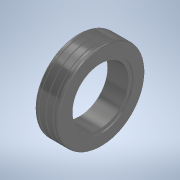
# Autodesk Inventor part: Wheel 75 mm - Part 1
Saved by Autodesk Inventor 2020 (Build 240168000, 168)
## iProperties
Created: 2023-01-26
Part Number: Wheel 75 mm - Part 1
Material: Generic
Document SubType Name: Modeling
Designer: saad.nashed
Density: 1 g/cm^3
Appearance: Rubber - Black - Version 1.1
d3: 24.000 mm
d4: 3.000 mm
d1: 20.250 mm
d5: 1.125 mm
d0: 37.500 mm
Author: saad.nashed
Autodesk Inventor part; units mm, degrees
ref_plane "YZ Plane" through (0, 0, 0) normal (1, 0, 0) x (0, 1, 0)
ref_plane "XZ Plane" through (0, 0, 0) normal (0, 1, 0) x (-1, 0, 0)
ref_plane "XY Plane" through (0, 0, 0) normal (0, 0, 1) x (1, 0, 0)
sketch "Sketch1" plane through (0, 0, 0) normal (0, 1, 0) x (-1, 0, 0)
  line L0 (13.955, 0) -> (0, 0) construction
  line L1 (0, 0) -> (0, -8.8012) construction
  line L2 (-9, -24) -> (9, -24)
  line L3 (9, -24) -> (9, -27)
  line L4 (9, -27) -> (10.125, -27)
  line L5 (10.125, -27) -> (10.125, -35.475)
  arc A0 (8.1, -37.5) -> (10.125, -35.475) centre (8.1, -35.475) ccw
  line L6 (8.1, -37.5) -> (-8.1, -37.5)
  arc A1 (-10.125, -35.475) -> (-8.1, -37.5) centre (-8.1, -35.475) ccw
  line L7 (-10.125, -35.475) -> (-10.125, -27)
  line L8 (-10.125, -27) -> (-9, -27)
  line L9 (-9, -27) -> (-9, -24)
  line L10 (7.3125, -37.5) -> (5.8125, -37.5)
  line L11 (5.8125, -37.5) -> (5.8125, -36.3)
  line L12 (5.8125, -36.3) -> (7.3125, -36.3)
  line L13 (7.3125, -36.3) -> (7.3125, -37.5)
  line L14 (0.75, -37.5) -> (-0.75, -37.5)
  line L15 (-0.75, -37.5) -> (-0.75, -36.3)
  line L16 (-0.75, -36.3) -> (0.75, -36.3)
  line L17 (0.75, -36.3) -> (0.75, -37.5)
  line L18 (-5.8125, -37.5) -> (-7.3125, -37.5)
  line L19 (-7.3125, -37.5) -> (-7.3125, -36.3)
  line L20 (-7.3125, -36.3) -> (-5.8125, -36.3)
  line L21 (-5.8125, -36.3) -> (-5.8125, -37.5)
  point P0 (-0.75, -37.5)
  dimension "d0" = 37.5
  dimension "d1" = 20.25
  dimension "d2" = 2.025
  dimension "d3" = 24
  dimension "d4" = 3
  dimension "d5" = 1.125
  dimension "d7" = 1.2
  dimension "d8" = 1.5
  dimension "d9" = 5.0625
  constraints: 44 end point, 10 perpendicular, 6 parallel, 5 horizontal, 4 point on circle, 4 point on line, 3 collinear, 3 symmetric about line, 3 tangent, 2 centre point, 6 other
  measures "d0" distance between parallel lines of L6 L0
  measures "d1" distance between parallel lines of L5 L7
  measures "d2" radius of A0
  measures "d3" distance between parallel lines of L2 L0
  measures "d4" distance between parallel lines of L4 L2
  measures "d5" distance between parallel lines of L5 L3
  measures "d7" distance between parallel lines of L6 L12
  measures "d8" distance between parallel lines of L11 L13
  measures "d9" distance between parallel lines of L17 L11
revolve "Revolution1" add sketch "Sketch1" angle 360 about axis through (-13.955, 0, 0) along (1, 0, 0) contours L2 L3 L4 L5 A0 L6 L13 L12 L11 L17 L16 L15 L21 L20 L19 A1 L7 L8 L9
equation "\"d1\" = 0.54 * d0"
equation "\"d2\" = 0.1 * d1"
equation "\"d3\" = 0.64 * d0"
equation "\"d4\" = 0.08 * d0"
equation "\"d5\" = 0.03 * d0"
equation "\"d9\" = 0.25 * d1"
body "Solid1"
